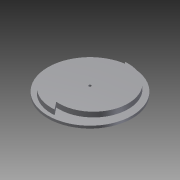
# Autodesk Inventor part: Rueda superior
Saved by Autodesk Inventor 2011 (Build 150239000, 239)
## iProperties
Created: 2014-08-04
Part Number: Rueda superior
Material: Por defecto
Document SubType Name: Chapa
Designer: amatiasq
Density: 1 g/cm^3
Sheet Metal Rule: Por defecto_mm
Author: amatiasq
Autodesk Inventor part; units mm, degrees
ref_plane "YZ Plane" through (0, 0, 0) normal (1, 0, 0) x (0, 1, 0)
ref_plane "XZ Plane" through (0, 0, 0) normal (0, 1, 0) x (-1, 0, 0)
ref_plane "XY Plane" through (0, 0, 0) normal (0, 0, 1) x (1, 0, 0)
sketch "Boceto1" plane through (0, 0, 0) normal (0, 0, 1) x (1, 0, 0)
  circle A0 centre (0, 0) radius 17
  circle A1 centre (0, 0) radius 0.5
  dimension "d0" = 34
  dimension "d1" = 1
  constraints: 2 centre point, 2 coincident
  measures "d0" diameter of A0
  measures "d1" diameter of A1
extrude "Extrusión1" add sketch "Boceto1" along normal blind 1
sketch "Boceto2" plane through (0, 0, 1) normal (0, 0, 1) x (1, 0, 0)
  circle A0 centre (0, 0) radius 0.5 projected
  arc A1 (0, -12.5) -> (0, 15.5) centre (-0.0655, 1.5) ccw
  arc A2 (-0.0312, 12.4605) -> (-0.0542, -15.5395) centre (-0.1439, -1.5394) ccw
  arc A3 (-0.0542, -15.5395) -> (1.1656, -15.4784) centre (-0.1439, -1.5398) ccw
  line L0 (-0.0542, -15.5395) -> (-0.1439, -1.5398) construction
  line L1 (1.1656, -15.4784) -> (-0.1439, -1.5398) construction
  arc A4 (-1.2204, -12.4524) -> (0, -12.5) centre (-0.0655, 1.4998) ccw
  line L2 (0, -12.5) -> (-0.0655, 1.4998) construction
  line L3 (-1.2204, -12.4524) -> (-0.0655, 1.4998) construction
  line L4 (-1.2204, -12.4524) -> (1.1656, -15.4784)
  arc A5 (1.1885, 12.3974) -> (-0.0312, 12.4605) centre (-0.1439, -1.5391) ccw
  line L5 (-0.0312, 12.4605) -> (-0.1439, -1.5391) construction
  line L6 (1.1885, 12.3974) -> (-0.1439, -1.5391) construction
  arc A6 (0, 15.5) -> (-1.2204, 15.4524) centre (-0.0655, 1.5002) ccw
  line L7 (0, 15.5) -> (-0.0655, 1.5002) construction
  line L8 (-1.2204, 15.4524) -> (-0.0655, 1.5002) construction
  line L9 (-1.2204, 15.4524) -> (1.1885, 12.3974)
  dimension "d4" = 28
  dimension "d5" = 28
  dimension "d6" = 14
  dimension "d7" = 5
  dimension "d8" = 14
  dimension "d9" = 5
  dimension "d10" = 14
  dimension "d11" = 5
  dimension "d12" = 14
  dimension "d13" = 5
  constraints: 20 end point, 12 point on circle, 6 centre point, 4 tangent, 1 parallel
  measures "d4" distance of L7.start L2.start
  measures "d5" distance of L0.start L5.start
  measures "d6" radius of A3
  measures "d7" angle of L0 L1
  measures "d8" radius of A4
  measures "d9" angle of L3 L2
  measures "d10" radius of A5
  measures "d11" angle of L6 L5
  measures "d12" radius of A6
  measures "d13" angle of L7 L8
extrude "Extrusión2" add sketch "Boceto2" along normal blind 2
equation "\"Radio_pliegue\" = Grosor"
equation "\"Anchura_desahogo_plegado\" = Grosor"
equation "\"Profundidad_desahogo_plegado\" = 0.5 * Grosor"
equation "\"Tamaño_destalonado\" = 4 * Grosor"
equation "\"Remanente_mínimo\" = 2 * Grosor"
equation "\"Radiodetransición\" = Radio_pliegue"
equation "\"Tamaño_de_radio_de_Jacobi\" = Radio_pliegue"
equation "\"TamañoSeparación\" = Grosor"
equation "\"Grosor\" = 0.5"
